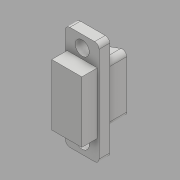
# Autodesk Inventor part: 15pin female connector
Saved by Autodesk Inventor 2017 (Build 210142000, 142)
## iProperties
Created: 2017-02-21
Part Number: 15pin female connector
Material: Generic
Document SubType Name: Modeling
Designer: qupec
Density: 1 g/cm^3
Appearance: Default
Author: qupec
Autodesk Inventor part; units mm, degrees
ref_plane "YZ Plane" through (0, 0, 0) normal (1, 0, 0) x (0, 1, 0)
ref_plane "XZ Plane" through (0, 0, 0) normal (0, 1, 0) x (-1, 0, 0)
ref_plane "XY Plane" through (0, 0, 0) normal (0, 0, 1) x (1, 0, 0)
sketch "Sketch1" plane through (0, 0, 0) normal (0, 1, 0) x (-1, 0, 0)
  line L0 (3.8, 11.75) -> (-3.8, 11.75)
  line L1 (-3.8, 11.75) -> (-3.8, -11.75)
  line L2 (-3.8, -11.75) -> (3.8, -11.75)
  line L3 (3.8, -11.75) -> (3.8, 11.75)
  circle A0 centre (0, 9.1) radius 1.6
  circle A1 centre (0, -9.1) radius 1.6
  point P0 (0, 0)
  dimension "d0" = 23.5
  dimension "d1" = 7.6
  dimension "d2" = 11.75
  dimension "d3" = 3.8
  dimension "d4" = 3.2
  dimension "d5" = 3.2
  dimension "d6" = 18.2
  dimension "d7" = 9.1
  constraints: 8 end point, 2 centre point, 2 parallel, 1 horizontal, 1 perpendicular
  measures "d0" distance of L2.end L0.start
  measures "d1" distance of L0.start L0.end
  measures "d2" distance from line of point (0, 0) L0
  measures "d3" distance from line of point (0, 0) L1
  measures "d4" diameter of A0
  measures "d5" diameter of A1
  measures "d6" distance of A1.centre A0.centre
  measures "d7" distance of point (0, 0) A0.centre
extrude "Extrusion1" add sketch "Sketch1" along normal blind 2.4
fillet "Fillet1" radius 1 4 edges at (3.8, 1.2, 11.75) (-3.8, 1.2, 11.75) (3.8, 1.2, -11.75) (-3.8, 1.2, -11.75)
sketch "Sketch2" plane through (0, 2.4, 0) normal (0, 1, 0) x (1, 0, 0)
  line L0 (-3.05, -4.6194) -> (-3.05, 4.6194)
  line L1 (-3.05, 4.6194) -> (3.05, 6.85)
  line L2 (3.05, 6.85) -> (3.05, -6.85)
  line L3 (3.05, -6.85) -> (-3.05, -4.6194)
  line L4 (2.55, -6.1348) -> (-2.55, -4.2698)
  line L5 (-2.55, -4.2698) -> (-2.55, 4.2698)
  line L6 (-2.55, 4.2698) -> (2.55, 6.1348)
  line L7 (2.55, 6.1348) -> (2.55, -6.1348)
  point P0 (0, 0)
  dimension "d11" = 69.914
  dimension "d13" = 13.7
  dimension "d14" = 6.1
  dimension "d15" = 3.05
  dimension "d17" = 0.5
  dimension "d18" = 0.5
  dimension "d19" = 0.5
  dimension "d20" = 0.5
  dimension "d21" = 6.85
  dimension "d22" = 69.914
  dimension "d23" = 69.914
  constraints: 16 end point, 3 parallel, 2 vertical
  measures "d11" angle of L2 L3
  measures "d13" distance of L1.end L2.end
  measures "d14" distance between parallel lines of L2 L0
  measures "d15" distance from line of L0 point (0, 0)
  measures "d17" distance between parallel lines of L0 L5
  measures "d18" distance between parallel lines of L3 L4
  measures "d19" distance between parallel lines of L2 L7
  measures "d20" distance between parallel lines of L1 L6
  measures "d21" vertical distance of point (0, 0) L2.end
  measures "d22" angle of L2 L1
  measures "d23" angle of L7 L4
extrude "Extrusion2" add sketch "Sketch2" along normal blind 4.6
fillet "Fillet2" radius 1 8 edges at (-3.05, 4.7, -4.6194) (-3.05, 4.7, 4.6194) (3.05, 4.7, 6.85) (3.05, 4.7, -6.85) (-2.55, 4.7, -4.2698) (-2.55, 4.7, 4.2698) (2.55, 4.7, -6.1348) (2.55, 4.7, 6.1348)
sketch "Sketch3" plane through (0, 0, 0) normal (0, -1, 0) x (1, 0, 0)
  line L0 (3.4, 6.9) -> (-3.4, 6.9)
  line L1 (-3.4, 6.9) -> (-3.4, -6.9)
  line L2 (-3.4, -6.9) -> (3.4, -6.9)
  line L3 (3.4, -6.9) -> (3.4, 6.9)
  point P0 (0, 0)
  dimension "d27" = 13.8
  dimension "d28" = 6.8
  dimension "d29" = 6.9
  dimension "d30" = 3.4
  constraints: 8 end point, 2 parallel, 1 horizontal, 1 perpendicular
  measures "d27" distance of L2.end L0.start
  measures "d28" distance of L1.end L2.end
  measures "d29" distance from line of point (0, 0) L2
  measures "d30" distance from line of point (0, 0) L3
extrude "Extrusion3" add sketch "Sketch3" along normal blind 3.5
equation "\"d2\" = 0.5 * d0"
equation "\"d3\" = 0.5 * d1"
equation "\"d5\" = d4"
equation "\"d7\" = 0.5 * d6"
equation "\"d15\" = 0.5 * d14"
equation "\"d21\" = 0.5 * d13"
equation "\"d22\" = d11"
equation "\"d29\" = 0.5 * d27"
equation "\"d30\" = 0.5 * d28"
body "Solid1"
